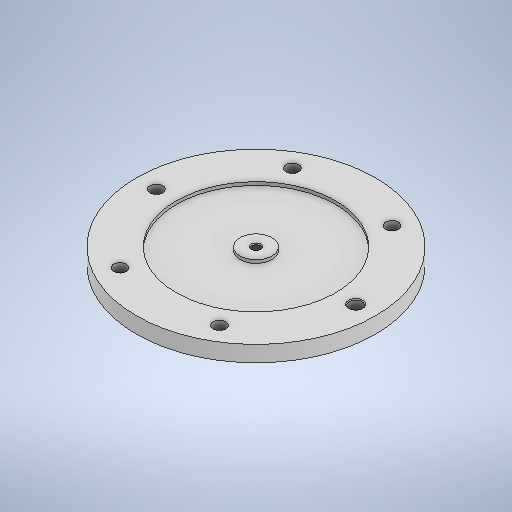
# Autodesk Inventor part: 10_Nap_cua_tham
Saved by Autodesk Inventor 2025.2 (Build 292293000, 293)
## iProperties
Created: 2024-11-27
Part Number: 10_Nap_cua_tham
Material: Generic
Document SubType Name: Modeling
Designer: hongquan
Density: 1 g/cm^3
Appearance: Default
Author: hongquan
Autodesk Inventor part; units mm, degrees
ref_plane "YZ Plane" through (0, 0, 0) normal (1, 0, 0) x (0, 1, 0)
ref_plane "XZ Plane" through (0, 0, 0) normal (0, 1, 0) x (-1, 0, 0)
ref_plane "XY Plane" through (0, 0, 0) normal (0, 0, 1) x (1, 0, 0)
sketch "Sketch1" plane through (0, 0, 0) normal (1, 0, 0) x (0, 1, 0)
  line L0 (2, 5) -> (9, 5)
  line L1 (9, 5) -> (9, 3)
  line L2 (9, 3) -> (10, 3)
  line L3 (10, 3) -> (10, 10)
  line L4 (10, 10) -> (8, 10)
  line L5 (8, 10) -> (8, 50)
  line L6 (8, 50) -> (10, 50)
  line L7 (10, 50) -> (10, 75)
  line L8 (10, 75) -> (0, 75)
  line L9 (0, 75) -> (0, 50)
  line L10 (0, 50) -> (2, 50)
  line L11 (2, 50) -> (2, 5)
  line L12 (24.985, 0) -> (-21.0801, 0)
  line L13 (0, 63.0325) -> (0, -71.2298) construction
  point P0 (0, 0)
  point P1 (5.5, 5)
  point P2 (5, 75)
  dimension "d0" = 150
  dimension "d1" = 10
  dimension "d2" = 2
  dimension "d3" = 7
  dimension "d4" = 1
  dimension "d5" = 7
  dimension "d6" = 2
  dimension "d7" = 25
  dimension "d8" = 47
  dimension "d9" = 0
  dimension "d10" = 70
  constraints: 28 end point, 9 perpendicular, 4 horizontal, 2 midpoint, 2 point on line, 2 vertical
  measures "d0" diameter of L8 L12
  measures "d1" distance of L7.end L8.end
  measures "d2" distance of L9.end L10.end
  measures "d3" distance of L0.start L0.end
  measures "d4" distance of L1.end L2.end
  measures "d5" distance of L2.end L3.end
  measures "d6" distance of L5.end L6.end
  measures "d7" distance of L6.end L7.end
  measures "d8" distance between parallel lines of L2 L6
  measures "d9" distance between parallel lines of L13 L9
  measures "d10" vertical distance of point (5.5, 5) point (5, 75)
revolve "Revolution1" add sketch "Sketch1" angle 360 about axis through (0, 24.985, 0) along (0, -1, 0)
sketch "Sketch2" plane through (0, 2, 0) normal (0, -1, 0) x (1, 0, 0)
  point P0 (0, 0)
sketch "Sketch3" plane through (0, 0, 0) normal (0, -1, 0) x (1, 0, 0)
  circle A0 centre (0, 0) radius 62.5
  circle A1 centre (62.5, 0) radius 4
  dimension "d12" = 125
  dimension "d13" = 8
  constraints: 2 coincident, 2 horizontal alignment, 1 centre point, 2 other
  measures "d13" diameter of A1
hole "Hole1" at (62.5, 0, 0) direction (0, 1, 0) diameter 8 end through all
chamfer "Chamfer1" distance 0.5 angle 45 1 edges at (62.5, 10, 4)
pattern_circular "Circular Pattern1" count 6 over 360 about axis through (0, 5, 0) along (0, -1, 0) of "Hole1"
body "Solid1"
